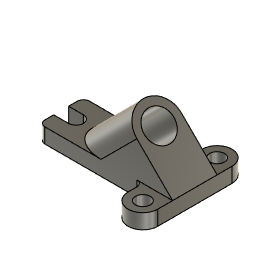
Part 14 (Autodesk Fusion 360 design; units mm, degrees)
Autodesk Fusion 360 part; units mm, degrees
sketch "Sketch7" plane through (0, 0, 0) normal (0, 0, 1) x (1, 0, 0)
  line L0 (-40, 7.5) -> (-5, 7.5)
  line L1 (-5, 7.5) -> (-5, 12.5)
  arc A0 (5, 12.5) -> (-5, 12.5) centre (0, 12.5) ccw
  line L2 (5, 12.5) -> (5, -12.5)
  arc A1 (-5, -12.5) -> (5, -12.5) centre (0, -12.5) ccw
  line L3 (-5, -12.5) -> (-5, -7.5)
  line L4 (-5, -7.5) -> (-40, -7.5)
  line L5 (-40, 2.5) -> (-35, 2.5)
  arc A2 (-35, -2.5) -> (-35, 2.5) centre (-35, 0) ccw
  line L6 (-35, -2.5) -> (-40, -2.5)
  line L7 (-40, -7.5) -> (-40, -2.5)
  line L8 (-40, 2.5) -> (-40, 7.5)
  circle A3 centre (0, 12.5) radius 2.5
  circle A4 centre (0, -12.5) radius 2.5
  dimension "d41" = 5
  dimension "d42" = 5
  dimension "d43" = 25
  dimension "d44" = 45
  dimension "d45" = 2.5
  dimension "d46" = 5
  dimension "d47" = 5
  dimension "d48" = 12.5
  dimension "d49" = 5
  dimension "d50" = 5
  constraint horizontal L0
  constraint perpendicular L0 L1
  constraint tangent L1 A0
  constraint tangent A0 L2
  constraint parallel L1 L2
  constraint tangent L2 A1
  constraint tangent A1 L3
  constraint parallel L2 L3
  constraint perpendicular L2 L4
  constraint perpendicular L0 L7
  constraint equal A0 A1
  constraint equal L1 L3
  constraint coincident L5.start L7
  constraint perpendicular L5 L7
  constraint tangent L5 A2
  constraint tangent A2 L6
  constraint perpendicular L6 L7
  constraint collinear L7 L8
  constraint equal L7 L8
  constraint concentric A0 A3
  constraint concentric A1 A4
  measures "d41" radius of A0
  measures "d42" distance of A1.start L3.end
  measures "d43" distance of A0.start L2.end
  measures "d44" distance of L2 L7
  measures "d45" radius of A2
  measures "d46" distance of L5.start L5.end
  measures "d47" distance of origin L2
  measures "d48" distance of origin A1.centre
  measures "d49" diameter of A3
  measures "d50" diameter of A4
extrude "Extrude6" add sketch "Sketch7" along normal blind 5
fillet "Fillet3" radius 2 4 edges at (-40, -7.5, 2.5) (-40, 7.5, 2.5) (-5, 7.5, 2.5) (-5, -7.5, 2.5)
ref_plane "WorkPlane3" through (5, 0, 5) normal (0.707107, 0, 0.707107) x (0, 1, 0)
sketch "Sketch8" plane through (5, 0, 5) normal (0.707107, 0, 0.707107) x (0, 1, 0)
  line L0 (-7.5, 0) -> (7.5, 0)
  line L1 (7.5, 0) -> (7.5, 17)
  line L2 (-7.5, 0) -> (-7.5, 17)
  arc A0 (7.5, 17) -> (-7.5, 17) centre (0, 17) ccw
  dimension "d55" = 7.5
  dimension "d56" = 17
  dimension "d57" = 17
  constraint horizontal L0
  constraint perpendicular L0 L1
  constraint perpendicular L0 L2
  constraint tangent L2 A0
  constraint equal L1 L2
  measures "d55" radius of A0
  measures "d56" distance of origin A0.centre
  measures "d57" distance of L0.end L1.end
extrude "Extrude7" add sketch "Sketch8" along normal up to surface end surface through (0, 0, 5) normal (0, 0, 1) offset 0
sketch "Sketch9" plane through (5, 0, 5) normal (0.707107, 0, 0.707107) x (0, 1, 0)
  line L0 (-7.5, 0) -> (7.5, 0)
  line L1 (7.5, 0) -> (7.5, 17)
  arc A0 (7.5, 17) -> (-7.5, 17) centre (0, 17) ccw
  line L2 (-7.5, 17) -> (-7.5, 0)
  circle A1 centre (0, 17) radius 3.75
  dimension "d60" = 7.5
  constraint concentric A0 A1
  measures "d60" diameter of A1
hole "Hole1" at (-7.0208, 0, 17.0208) direction (-0.707107, 0, -0.707107) diameter 10 depth 17 tip angle 118
